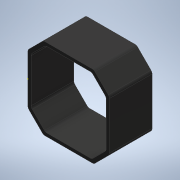
# Autodesk Inventor part: Part2
Saved by Autodesk Inventor 2021 (Build 250183000, 183)
## iProperties
Created: 2020-06-30
Part Number: Part2
Material: Genérico
Document SubType Name: Modeling
Designer: IVAN
Density: 1 g/cm^3
Appearance: Por defecto
Author: IVAN
Autodesk Inventor part; units mm, degrees
ref_plane "YZ Plane" through (0, 0, 0) normal (1, 0, 0) x (0, 1, 0)
ref_plane "XZ Plane" through (0, 0, 0) normal (0, 1, 0) x (-1, 0, 0)
ref_plane "XY Plane" through (0, 0, 0) normal (0, 0, 1) x (1, 0, 0)
sketch "Sketch1" plane through (0, 0, 0) normal (0, 1, 0) x (-1, 0, 0)
  line L0 (21, -21) -> (-21, -21)
  line L1 (-21, -21) -> (-21, 21)
  line L2 (-21, 21) -> (21, 21)
  line L3 (21, 21) -> (21, -21)
  line L4 (21, -21) -> (-21, 21) construction
  line L5 (-21, -21) -> (21, 21) construction
  point P0 (0, 0)
  dimension "d0" = 42
  dimension "d1" = 42
  constraints: 12 end point, 2 midpoint, 2 parallel, 1 horizontal, 1 perpendicular
  measures "d0" distance of L1.end L2.end
  measures "d1" distance of L0.end L1.end
extrude "Extrusion1" add sketch "Sketch1" along normal blind 22
chamfer "Chamfer1" distance 8 angle 45 4 edges at (21, 11, 21) (-21, 11, 21) (-21, 11, -21) (21, 11, -21)
fillet "Fillet1" radius 2 8 edges at (-13, 11, -21) (-21, 11, -13) (-21, 11, 13) (-13, 11, 21) (13, 11, 21) (21, 11, 13) (13, 11, -21) (21, 11, -13)
sketch "Sketch4" plane through (0, 22, 0) normal (0, 1, 0) x (1, 0, 0)
  arc A0 (21, 12.1716) -> (20.4142, 13.5858) centre (19, 12.1716) ccw projected
  line L0 (13.5858, 20.4142) -> (20.4142, 13.5858) projected
  arc A1 (13.5858, 20.4142) -> (12.1716, 21) centre (12.1716, 19) ccw projected
  line L1 (12.1716, 21) -> (-12.1716, 21) projected
  arc A2 (-12.1716, 21) -> (-13.5858, 20.4142) centre (-12.1716, 19) ccw projected
  line L2 (-20.4142, 13.5858) -> (-13.5858, 20.4142) projected
  arc A3 (-20.4142, 13.5858) -> (-21, 12.1716) centre (-19, 12.1716) ccw projected
  line L3 (-21, 12.1716) -> (-21, -12.1716) projected
  arc A4 (-21, -12.1716) -> (-20.4142, -13.5858) centre (-19, -12.1716) ccw projected
  line L4 (-13.5858, -20.4142) -> (-20.4142, -13.5858) projected
  arc A5 (-13.5858, -20.4142) -> (-12.1716, -21) centre (-12.1716, -19) ccw projected
  line L5 (-12.1716, -21) -> (12.1716, -21) projected
  arc A6 (12.1716, -21) -> (13.5858, -20.4142) centre (12.1716, -19) ccw projected
  line L6 (20.4142, -13.5858) -> (13.5858, -20.4142) projected
  arc A7 (20.4142, -13.5858) -> (21, -12.1716) centre (19, -12.1716) ccw projected
  line L7 (21, -12.1716) -> (21, 12.1716) projected
  arc A8 (19.32, 11.1978) -> (18.7811, 12.4989) centre (17.48, 11.1978) ccw
  line L8 (12.4989, 18.7811) -> (18.7811, 12.4989)
  arc A9 (12.4989, 18.7811) -> (11.1978, 19.32) centre (11.1978, 17.48) ccw
  line L9 (11.1978, 19.32) -> (-11.1978, 19.32)
  arc A10 (-11.1978, 19.32) -> (-12.4989, 18.7811) centre (-11.1978, 17.48) ccw
  line L10 (-18.7811, 12.4989) -> (-12.4989, 18.7811)
  arc A11 (-18.7811, 12.4989) -> (-19.32, 11.1978) centre (-17.48, 11.1978) ccw
  line L11 (-19.32, 11.1978) -> (-19.32, -11.1978)
  arc A12 (-19.32, -11.1978) -> (-18.7811, -12.4989) centre (-17.48, -11.1978) ccw
  line L12 (-12.4989, -18.7811) -> (-18.7811, -12.4989)
  arc A13 (-12.4989, -18.7811) -> (-11.1978, -19.32) centre (-11.1978, -17.48) ccw
  line L13 (-11.1978, -19.32) -> (11.1978, -19.32)
  arc A14 (11.1978, -19.32) -> (12.4989, -18.7811) centre (11.1978, -17.48) ccw
  line L14 (18.7811, -12.4989) -> (12.4989, -18.7811)
  arc A15 (18.7811, -12.4989) -> (19.32, -11.1978) centre (17.48, -11.1978) ccw
  line L15 (19.32, -11.1978) -> (19.32, 11.1978)
  point P0 (0, 0)
  point P1 (0, 0)
  constraints: 16 end point, 16 point on circle, 8 centre point
extrude "Extrusion2" cut sketch "Sketch4" against normal up to surface (22 mm away) contours L15 A15 L14 A14 L13 A13 L12 A12 L11 A11 L10 A10 L9 A9 L8 A8
sketch "Sketch5" plane through (-21, 0, -12.1716) normal (-1, 0, 0) x (0, 0, 1)
  line L0 (2.1716, 15.3239) -> (22.1716, 15.3239)
  line L1 (22.1716, 15.3239) -> (22.1716, 5.3239)
  line L2 (22.1716, 5.3239) -> (2.1716, 5.3239)
  line L3 (2.1716, 5.3239) -> (2.1716, 15.3239)
  line L4 (2.1716, 15.3239) -> (22.1716, 5.3239) construction
  line L5 (22.1716, 15.3239) -> (2.1716, 5.3239) construction
  point P0 (12.1716, 0)
  point P1 (12.1716, 10.3239)
  dimension "d18" = 20
  dimension "d19" = 10
  dimension "d20" = 10
  constraints: 12 end point, 2 midpoint, 2 parallel, 1 horizontal, 1 perpendicular
  measures "d18" distance of L0.start L0.end
  measures "d19" distance of L0.end L1.end
  measures "d20" distance from line of point (12.172, 0) L3
extrude "Extrusion3" add sketch "Sketch5" along normal blind 0.001
sketch "Sketch6" plane through (-21.001, 0, -12.1716) normal (-1, 0, 0) x (0, 0, 1)
  line L0 (2.7184, 14.6945) -> (21.7293, 14.6945) construction
  line L1 (21.7293, 14.6945) -> (21.7293, 6.3236) construction
  line L2 (21.7293, 6.3236) -> (2.7184, 6.3236) construction
  line L3 (2.7184, 6.3236) -> (2.7184, 14.6945) construction
  point P0 (12.1716, 0)
  constraints: 2 other
fillet "Fillet2" radius 2 4 edges at (-21.0005, 15.3239, -10) (-21.0005, 5.3239, -10) (-21.0005, 5.3239, 10) (-21.0005, 15.3239, 10)
body "Solid1"
